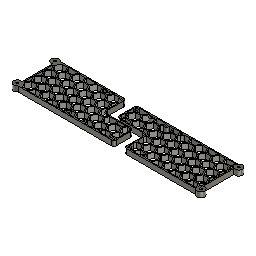
ERCP_Array_Support_Plate_350 (Autodesk Fusion 360 design; units mm, degrees)
Autodesk Fusion 360 part; units mm, degrees
(part 1 of 2)
sketch "Sketch1" plane through (0, 0, 0) normal (0, 0, 1) x (1, 0, 0)
  line L0 (0, 0) -> (490, 0) construction
  line L1 (490, 0) -> (490, 101) construction
  line L2 (490, 101) -> (0, 101) construction
  line L3 (0, 101) -> (0, 0) construction
  circle A0 centre (0, 101) radius 10
  circle A1 centre (0, 0) radius 10
  circle A2 centre (490, 101) radius 10
  circle A3 centre (490, 0) radius 10
  line L4 (0, 50.5) -> (490, 50.5) construction
  circle A4 centre (137.5, 101) radius 2.175
  circle A5 centre (137.5, 101) radius 6
  line L5 (0, 50.5) -> (23.3827, 37) construction
  line L6 (0, 50.5) -> (36.3739, 50.5) construction
  line L7 (23.3827, 37) -> (0, 23.5) construction
  line L8 (23.3827, 37) -> (42.9186, 37) construction
  line L9 (0, 23.5) -> (23.3827, 10) construction
  line L10 (0, 23.5) -> (20, 23.5) construction
  line L11 (211.5, 101) -> (211.5, 63)
  line L12 (263.5, 0) -> (263.5, 38)
  line L13 (183.5, 101) -> (183.5, 58)
  line L14 (291.5, 43) -> (291.5, 0)
  circle A6 centre (0, 0) radius 3
  circle A7 centre (0, 101) radius 3
  circle A8 centre (490, 0) radius 3
  circle A9 centre (490, 101) radius 3
  line L15 (8, 107) -> (177.5, 107)
  line L16 (217.5, 107) -> (482, 107)
  line L17 (482, -6) -> (297.5, -6)
  line L18 (257.5, -6) -> (8, -6)
  line L19 (221.5, 53) -> (281.5, 53)
  line L20 (193.5, 48) -> (253.5, 48)
  arc A10 (183.5, 58) -> (193.5, 48) centre (193.5, 58) ccw
  arc A11 (211.5, 63) -> (221.5, 53) centre (221.5, 63) ccw
  arc A12 (291.5, 43) -> (281.5, 53) centre (281.5, 43) ccw
  arc A13 (263.5, 38) -> (253.5, 48) centre (253.5, 38) ccw
  circle A14 centre (137.5, 0) radius 6
  circle A15 centre (137.5, 0) radius 2.175
  circle A16 centre (177.5, 101) radius 6
  circle A17 centre (177.5, 101) radius 2.175
  circle A18 centre (217.5, 101) radius 6
  circle A19 centre (217.5, 101) radius 2.175
  circle A20 centre (257.5, 101) radius 6
  circle A21 centre (257.5, 101) radius 2.175
  circle A22 centre (297.5, 101) radius 6
  circle A23 centre (297.5, 101) radius 2.175
  circle A24 centre (337.5, 101) radius 6
  circle A25 centre (337.5, 101) radius 2.175
  circle A26 centre (177.5, 0) radius 6
  circle A27 centre (177.5, 0) radius 2.175
  circle A28 centre (217.5, 0) radius 6
  circle A29 centre (217.5, 0) radius 2.175
  circle A30 centre (257.5, 0) radius 6
  circle A31 centre (257.5, 0) radius 2.175
  circle A32 centre (297.5, 0) radius 6
  circle A33 centre (297.5, 0) radius 2.175
  circle A34 centre (337.5, 0) radius 6
  circle A35 centre (337.5, 0) radius 2.175
  line L21 (181, 101) -> (181, 58)
  arc A36 (181, 58) -> (193.5, 45.5) centre (193.5, 58) ccw
  line L22 (193.5, 45.5) -> (253.5, 45.5)
  arc A37 (261, 38) -> (253.5, 45.5) centre (253.5, 38) ccw
  line L23 (261, 0) -> (261, 38)
  line L24 (214, 101) -> (214, 63)
  arc A38 (214, 63) -> (221.5, 55.5) centre (221.5, 63) ccw
  line L25 (221.5, 55.5) -> (281.5, 55.5)
  arc A39 (294, 43) -> (281.5, 55.5) centre (281.5, 43) ccw
  line L26 (294, 43) -> (294, 0)
  line L27 (8, 104.5) -> (177.5, 104.5)
  line L28 (257.5, -3.5) -> (8, -3.5)
  line L29 (482, -3.5) -> (297.5, -3.5)
  line L30 (217.5, 104.5) -> (482, 104.5)
  line L31 (6.9282, 38.5) -> (13.8564, 50.5)
  line L32 (13.8564, 50.5) -> (6.9282, 62.5)
  line L33 (6.9282, 62.5) -> (-6.9282, 62.5)
  line L34 (-6.9282, 62.5) -> (-13.8564, 50.5)
  line L35 (-13.8564, 50.5) -> (-6.9282, 38.5)
  line L36 (-6.9282, 38.5) -> (6.9282, 38.5)
  line L37 (30.3109, 25) -> (37.2391, 37)
  line L38 (37.2391, 37) -> (30.3109, 49)
  line L39 (30.3109, 49) -> (16.4545, 49)
  line L40 (16.4545, 49) -> (9.5263, 37)
  line L41 (9.5263, 37) -> (16.4545, 25)
  line L42 (16.4545, 25) -> (30.3109, 25)
  line L43 (-6.9282, 35.5) -> (-13.8564, 23.5)
  line L44 (-13.8564, 23.5) -> (-6.9282, 11.5)
  line L45 (-6.9282, 11.5) -> (6.9282, 11.5)
  line L46 (6.9282, 11.5) -> (13.8564, 23.5)
  line L47 (13.8564, 23.5) -> (6.9282, 35.5)
  line L48 (6.9282, 35.5) -> (-6.9282, 35.5)
  line L49 (16.4545, 22) -> (9.5263, 10)
  line L50 (9.5263, 10) -> (16.4545, -2)
  line L51 (16.4545, -2) -> (30.3109, -2)
  line L52 (30.3109, -2) -> (37.2391, 10)
  line L53 (37.2391, 10) -> (30.3109, 22)
  line L54 (30.3109, 22) -> (16.4545, 22)
  line L55 (6.9282, 65.5) -> (13.8564, 77.5)
  line L56 (13.8564, 77.5) -> (6.9282, 89.5)
  line L57 (6.9282, 89.5) -> (-6.9282, 89.5)
  line L58 (-6.9282, 89.5) -> (-13.8564, 77.5)
  line L59 (-13.8564, 77.5) -> (-6.9282, 65.5)
  line L60 (-6.9282, 65.5) -> (6.9282, 65.5)
  line L61 (3, 101) -> (3, 0)
  line L62 (487, 101) -> (487, 0)
  line L63 (484, 101) -> (484, 0)
  line L64 (6, 101) -> (6, 0)
  line L65 (137.5, 101) -> (137.5, 146) construction
  line L66 (145, 131) -> (130, 131) construction
  line L67 (130, 131) -> (130, 161) construction
  line L68 (130, 161) -> (145, 161) construction
  line L69 (145, 161) -> (145, 131) construction
  line L70 (145, 131) -> (130, 161) construction
  line L71 (130, 131) -> (145, 161) construction
  line L72 (125, 161) -> (165, 161) construction
  line L73 (165, 161) -> (165, 131) construction
  line L74 (165, 131) -> (125, 131) construction
  line L75 (125, 131) -> (125, 161) construction
  line L76 (125, 181) -> (365, 181) construction
  line L77 (365, 181) -> (365, 151) construction
  line L78 (365, 151) -> (125, 151) construction
  line L79 (125, 151) -> (125, 181) construction
  line L80 (245, 181) -> (245, 151) construction
  line L81 (32.909, 23.5) -> (39.8372, 11.5)
  line L82 (39.8372, 35.5) -> (32.909, 23.5)
  line L83 (53.6936, 35.5) -> (39.8372, 35.5)
  line L84 (60.6218, 23.5) -> (53.6936, 35.5)
  line L85 (53.6936, 11.5) -> (60.6218, 23.5)
  line L86 (63.2199, 22) -> (56.2917, 10)
  line L87 (39.8372, 11.5) -> (53.6936, 11.5)
  line L88 (53.6936, 8.5) -> (39.8372, 8.5)
  line L89 (60.6218, -3.5) -> (53.6936, 8.5)
  line L90 (53.6936, -15.5) -> (60.6218, -3.5)
  line L91 (39.8372, -15.5) -> (53.6936, -15.5)
  line L92 (32.909, -3.5) -> (39.8372, -15.5)
  line L93 (39.8372, 8.5) -> (32.909, -3.5)
  line L94 (77.0763, 22) -> (63.2199, 22)
  line L95 (56.2917, 10) -> (63.2199, -2)
  line L96 (63.2199, -2) -> (77.0763, -2)
  line L97 (77.0763, -2) -> (84.0045, 10)
  line L98 (84.0045, 10) -> (77.0763, 22)
  line L99 (77.0763, -5) -> (63.2199, -5)
  line L100 (63.2199, -5) -> (56.2917, -17)
  line L101 (56.2917, -17) -> (63.2199, -29)
  line L102 (63.2199, -29) -> (77.0763, -29)
  line L103 (77.0763, -29) -> (84.0045, -17)
  line L104 (84.0045, -17) -> (77.0763, -5)
  line L105 (79.6743, -3.5) -> (86.6025, -15.5)
  line L106 (86.6025, 8.5) -> (79.6743, -3.5)
  line L107 (100.4589, 8.5) -> (86.6025, 8.5)
  line L108 (107.3872, -3.5) -> (100.4589, 8.5)
  line L109 (100.4589, -15.5) -> (107.3872, -3.5)
  line L110 (109.9852, -5) -> (103.057, -17)
  line L111 (86.6025, -15.5) -> (100.4589, -15.5)
  line L112 (100.4589, -18.5) -> (86.6025, -18.5)
  line L113 (107.3872, -30.5) -> (100.4589, -18.5)
  line L114 (100.4589, -42.5) -> (107.3872, -30.5)
  line L115 (86.6025, -42.5) -> (100.4589, -42.5)
  line L116 (79.6743, -30.5) -> (86.6025, -42.5)
  line L117 (86.6025, -18.5) -> (79.6743, -30.5)
  line L118 (123.8416, -5) -> (109.9852, -5)
  line L119 (103.057, -17) -> (109.9852, -29)
  line L120 (109.9852, -29) -> (123.8416, -29)
  line L121 (123.8416, -29) -> (130.7698, -17)
  line L122 (130.7698, -17) -> (123.8416, -5)
  line L123 (123.8416, -32) -> (109.9852, -32)
  line L124 (109.9852, -32) -> (103.057, -44)
  line L125 (103.057, -44) -> (109.9852, -56)
  line L126 (109.9852, -56) -> (123.8416, -56)
  line L127 (123.8416, -56) -> (130.7698, -44)
  line L128 (130.7698, -44) -> (123.8416, -32)
  line L129 (126.4397, -30.5) -> (133.3679, -42.5)
  line L130 (133.3679, -18.5) -> (126.4397, -30.5)
  line L131 (147.2243, -18.5) -> (133.3679, -18.5)
  line L132 (154.1525, -30.5) -> (147.2243, -18.5)
  line L133 (147.2243, -42.5) -> (154.1525, -30.5)
  line L134 (156.7506, -32) -> (149.8224, -44)
  line L135 (133.3679, -42.5) -> (147.2243, -42.5)
  line L136 (147.2243, -45.5) -> (133.3679, -45.5)
  line L137 (154.1525, -57.5) -> (147.2243, -45.5)
  line L138 (147.2243, -69.5) -> (154.1525, -57.5)
  line L139 (133.3679, -69.5) -> (147.2243, -69.5)
  line L140 (126.4397, -57.5) -> (133.3679, -69.5)
  line L141 (133.3679, -45.5) -> (126.4397, -57.5)
  line L142 (170.607, -32) -> (156.7506, -32)
  line L143 (149.8224, -44) -> (156.7506, -56)
  line L144 (156.7506, -56) -> (170.607, -56)
  line L145 (170.607, -56) -> (177.5352, -44)
  line L146 (177.5352, -44) -> (170.607, -32)
  line L147 (170.607, -59) -> (156.7506, -59)
  line L148 (156.7506, -59) -> (149.8224, -71)
  line L149 (149.8224, -71) -> (156.7506, -83)
  line L150 (156.7506, -83) -> (170.607, -83)
  line L151 (170.607, -83) -> (177.5352, -71)
  line L152 (177.5352, -71) -> (170.607, -59)
  line L153 (173.2051, -57.5) -> (180.1333, -69.5)
  line L154 (180.1333, -45.5) -> (173.2051, -57.5)
  line L155 (193.9897, -45.5) -> (180.1333, -45.5)
  line L156 (200.9179, -57.5) -> (193.9897, -45.5)
  line L157 (193.9897, -69.5) -> (200.9179, -57.5)
  line L158 (203.516, -59) -> (196.5878, -71)
  line L159 (180.1333, -69.5) -> (193.9897, -69.5)
  line L160 (193.9897, -72.5) -> (180.1333, -72.5)
  line L161 (200.9179, -84.5) -> (193.9897, -72.5)
  line L162 (193.9897, -96.5) -> (200.9179, -84.5)
  line L163 (180.1333, -96.5) -> (193.9897, -96.5)
  line L164 (173.2051, -84.5) -> (180.1333, -96.5)
  line L165 (180.1333, -72.5) -> (173.2051, -84.5)
  line L166 (217.3724, -59) -> (203.516, -59)
  line L167 (196.5878, -71) -> (203.516, -83)
  line L168 (203.516, -83) -> (217.3724, -83)
  line L169 (217.3724, -83) -> (224.3006, -71)
  line L170 (224.3006, -71) -> (217.3724, -59)
  line L171 (217.3724, -86) -> (203.516, -86)
  line L172 (203.516, -86) -> (196.5878, -98)
  line L173 (196.5878, -98) -> (203.516, -110)
  line L174 (203.516, -110) -> (217.3724, -110)
  line L175 (217.3724, -110) -> (224.3006, -98)
  line L176 (224.3006, -98) -> (217.3724, -86)
  line L177 (219.9705, -84.5) -> (226.8987, -96.5)
  line L178 (226.8987, -72.5) -> (219.9705, -84.5)
  line L179 (240.7551, -72.5) -> (226.8987, -72.5)
  line L180 (247.6833, -84.5) -> (240.7551, -72.5)
  line L181 (240.7551, -96.5) -> (247.6833, -84.5)
  line L182 (250.2813, -86) -> (243.3531, -98)
  line L183 (226.8987, -96.5) -> (240.7551, -96.5)
  line L184 (240.7551, -99.5) -> (226.8987, -99.5)
  line L185 (247.6833, -111.5) -> (240.7551, -99.5)
  line L186 (240.7551, -123.5) -> (247.6833, -111.5)
  line L187 (226.8987, -123.5) -> (240.7551, -123.5)
  line L188 (219.9705, -111.5) -> (226.8987, -123.5)
  line L189 (226.8987, -99.5) -> (219.9705, -111.5)
  line L190 (264.1377, -86) -> (250.2813, -86)
  line L191 (243.3531, -98) -> (250.2813, -110)
  line L192 (250.2813, -110) -> (264.1377, -110)
  line L193 (264.1377, -110) -> (271.066, -98)
  line L194 (271.066, -98) -> (264.1377, -86)
  line L195 (264.1377, -113) -> (250.2813, -113)
  line L196 (250.2813, -113) -> (243.3531, -125)
  line L197 (243.3531, -125) -> (250.2813, -137)
  line L198 (250.2813, -137) -> (264.1377, -137)
  line L199 (264.1377, -137) -> (271.066, -125)
  line L200 (271.066, -125) -> (264.1377, -113)
  line L201 (266.7358, -111.5) -> (273.664, -123.5)
  line L202 (273.664, -99.5) -> (266.7358, -111.5)
  line L203 (287.5204, -99.5) -> (273.664, -99.5)
  line L204 (294.4486, -111.5) -> (287.5204, -99.5)
  line L205 (287.5204, -123.5) -> (294.4486, -111.5)
  line L206 (297.0467, -113) -> (290.1185, -125)
  line L207 (273.664, -123.5) -> (287.5204, -123.5)
  line L208 (287.5204, -126.5) -> (273.664, -126.5)
  line L209 (294.4486, -138.5) -> (287.5204, -126.5)
  line L210 (287.5204, -150.5) -> (294.4486, -138.5)
  line L211 (273.664, -150.5) -> (287.5204, -150.5)
  line L212 (266.7358, -138.5) -> (273.664, -150.5)
  line L213 (273.664, -126.5) -> (266.7358, -138.5)
  line L214 (310.9031, -113) -> (297.0467, -113)
  line L215 (290.1185, -125) -> (297.0467, -137)
  line L216 (297.0467, -137) -> (310.9031, -137)
  line L217 (310.9031, -137) -> (317.8313, -125)
  line L218 (317.8313, -125) -> (310.9031, -113)
  line L219 (310.9031, -140) -> (297.0467, -140)
  line L220 (297.0467, -140) -> (290.1185, -152)
  line L221 (290.1185, -152) -> (297.0467, -164)
  line L222 (297.0467, -164) -> (310.9031, -164)
  line L223 (310.9031, -164) -> (317.8313, -152)
  line L224 (317.8313, -152) -> (310.9031, -140)
  line L225 (313.5012, -138.5) -> (320.4294, -150.5)
  line L226 (320.4294, -126.5) -> (313.5012, -138.5)
  line L227 (334.2858, -126.5) -> (320.4294, -126.5)
  line L228 (341.214, -138.5) -> (334.2858, -126.5)
  line L229 (334.2858, -150.5) -> (341.214, -138.5)
  line L230 (343.8121, -140) -> (336.8839, -152)
  line L231 (320.4294, -150.5) -> (334.2858, -150.5)
  line L232 (334.2858, -153.5) -> (320.4294, -153.5)
  line L233 (341.214, -165.5) -> (334.2858, -153.5)
  line L234 (334.2858, -177.5) -> (341.214, -165.5)
  line L235 (320.4294, -177.5) -> (334.2858, -177.5)
  line L236 (313.5012, -165.5) -> (320.4294, -177.5)
  line L237 (320.4294, -153.5) -> (313.5012, -165.5)
  line L238 (357.6685, -140) -> (343.8121, -140)
  line L239 (336.8839, -152) -> (343.8121, -164)
  line L240 (343.8121, -164) -> (357.6685, -164)
  line L241 (357.6685, -164) -> (364.5967, -152)
  line L242 (364.5967, -152) -> (357.6685, -140)
  line L243 (357.6685, -167) -> (343.8121, -167)
  line L244 (343.8121, -167) -> (336.8839, -179)
  line L245 (336.8839, -179) -> (343.8121, -191)
  line L246 (343.8121, -191) -> (357.6685, -191)
  line L247 (357.6685, -191) -> (364.5967, -179)
  line L248 (364.5967, -179) -> (357.6685, -167)
  line L249 (360.2666, -165.5) -> (367.1948, -177.5)
  line L250 (367.1948, -153.5) -> (360.2666, -165.5)
  line L251 (381.0512, -153.5) -> (367.1948, -153.5)
  line L252 (387.9794, -165.5) -> (381.0512, -153.5)
  line L253 (381.0512, -177.5) -> (387.9794, -165.5)
  line L254 (390.5775, -167) -> (383.6493, -179)
  line L255 (367.1948, -177.5) -> (381.0512, -177.5)
  line L256 (381.0512, -180.5) -> (367.1948, -180.5)
  line L257 (387.9794, -192.5) -> (381.0512, -180.5)
  line L258 (381.0512, -204.5) -> (387.9794, -192.5)
  line L259 (367.1948, -204.5) -> (381.0512, -204.5)
  line L260 (360.2666, -192.5) -> (367.1948, -204.5)
  line L261 (367.1948, -180.5) -> (360.2666, -192.5)
  line L262 (404.4339, -167) -> (390.5775, -167)
  line L263 (383.6493, -179) -> (390.5775, -191)
  line L264 (390.5775, -191) -> (404.4339, -191)
  line L265 (404.4339, -191) -> (411.3621, -179)
  line L266 (411.3621, -179) -> (404.4339, -167)
  line L267 (404.4339, -194) -> (390.5775, -194)
  line L268 (390.5775, -194) -> (383.6493, -206)
  line L269 (383.6493, -206) -> (390.5775, -218)
  line L270 (390.5775, -218) -> (404.4339, -218)
  line L271 (404.4339, -218) -> (411.3621, -206)
  line L272 (411.3621, -206) -> (404.4339, -194)
  line L273 (9.5236, 90.9953) -> (16.4518, 78.9953)
  line L274 (16.4518, 102.9953) -> (9.5236, 90.9953)
  line L275 (30.3082, 102.9953) -> (16.4518, 102.9953)
  line L276 (37.2364, 90.9953) -> (30.3082, 102.9953)
  line L277 (30.3082, 78.9953) -> (37.2364, 90.9953)
  line L278 (39.8345, 89.4953) -> (32.9063, 77.4953)
  line L279 (16.4518, 78.9953) -> (30.3082, 78.9953)
  line L280 (30.3082, 75.9953) -> (16.4518, 75.9953)
  line L281 (37.2364, 63.9953) -> (30.3082, 75.9953)
  line L282 (30.3082, 51.9953) -> (37.2364, 63.9953)
  line L283 (16.4518, 51.9953) -> (30.3082, 51.9953)
  line L284 (9.5236, 63.9953) -> (16.4518, 51.9953)
  line L285 (16.4518, 75.9953) -> (9.5236, 63.9953)
  line L286 (53.6909, 89.4953) -> (39.8345, 89.4953)
  line L287 (32.9063, 77.4953) -> (39.8345, 65.4953)
  line L288 (39.8345, 65.4953) -> (53.6909, 65.4953)
  line L289 (53.6909, 65.4953) -> (60.6191, 77.4953)
  line L290 (60.6191, 77.4953) -> (53.6909, 89.4953)
  line L291 (53.6909, 62.4953) -> (39.8345, 62.4953)
  line L292 (39.8345, 62.4953) -> (32.9063, 50.4953)
  line L293 (32.9063, 50.4953) -> (39.8345, 38.4953)
  line L294 (39.8345, 38.4953) -> (53.6909, 38.4953)
  line L295 (53.6909, 38.4953) -> (60.6191, 50.4953)
  line L296 (60.6191, 50.4953) -> (53.6909, 62.4953)
  line L297 (56.289, 63.9953) -> (63.2172, 51.9953)
  line L298 (63.2172, 75.9953) -> (56.289, 63.9953)
  line L299 (77.0736, 75.9953) -> (63.2172, 75.9953)
  line L300 (84.0018, 63.9953) -> (77.0736, 75.9953)
  line L301 (77.0736, 51.9953) -> (84.0018, 63.9953)
  line L302 (86.5999, 62.4953) -> (79.6717, 50.4953)
  line L303 (63.2172, 51.9953) -> (77.0736, 51.9953)
  line L304 (77.0736, 48.9953) -> (63.2172, 48.9953)
  line L305 (84.0018, 36.9953) -> (77.0736, 48.9953)
  line L306 (77.0736, 24.9953) -> (84.0018, 36.9953)
  line L307 (63.2172, 24.9953) -> (77.0736, 24.9953)
  line L308 (56.289, 36.9953) -> (63.2172, 24.9953)
  line L309 (63.2172, 48.9953) -> (56.289, 36.9953)
  line L310 (100.4563, 62.4953) -> (86.5999, 62.4953)
  line L311 (79.6717, 50.4953) -> (86.5999, 38.4953)
  line L312 (86.5999, 38.4953) -> (100.4563, 38.4953)
  line L313 (100.4563, 38.4953) -> (107.3845, 50.4953)
  line L314 (107.3845, 50.4953) -> (100.4563, 62.4953)
  line L315 (100.4563, 35.4953) -> (86.5999, 35.4953)
  line L316 (86.5999, 35.4953) -> (79.6717, 23.4953)
  line L317 (79.6717, 23.4953) -> (86.5999, 11.4953)
  line L318 (86.5999, 11.4953) -> (100.4563, 11.4953)
  line L319 (100.4563, 11.4953) -> (107.3845, 23.4953)
  line L320 (107.3845, 23.4953) -> (100.4563, 35.4953)
  line L321 (103.0543, 36.9953) -> (109.9825, 24.9953)
  line L322 (109.9825, 48.9953) -> (103.0543, 36.9953)
  line L323 (123.8389, 48.9953) -> (109.9825, 48.9953)
  line L324 (130.7672, 36.9953) -> (123.8389, 48.9953)
  line L325 (123.8389, 24.9953) -> (130.7672, 36.9953)
  line L326 (133.3652, 35.4953) -> (126.437, 23.4953)
  line L327 (109.9825, 24.9953) -> (123.8389, 24.9953)
  line L328 (123.8389, 21.9953) -> (109.9825, 21.9953)
  line L329 (130.7672, 9.9953) -> (123.8389, 21.9953)
  line L330 (123.8389, -2.0047) -> (130.7672, 9.9953)
  line L331 (109.9825, -2.0047) -> (123.8389, -2.0047)
  line L332 (103.0543, 9.9953) -> (109.9825, -2.0047)
  line L333 (109.9825, 21.9953) -> (103.0543, 9.9953)
  line L334 (147.2216, 35.4953) -> (133.3652, 35.4953)
  line L335 (126.437, 23.4953) -> (133.3652, 11.4953)
  line L336 (133.3652, 11.4953) -> (147.2216, 11.4953)
  line L337 (147.2216, 11.4953) -> (154.1498, 23.4953)
  line L338 (154.1498, 23.4953) -> (147.2216, 35.4953)
  line L339 (147.2216, 8.4953) -> (133.3652, 8.4953)
  line L340 (133.3652, 8.4953) -> (126.437, -3.5047)
  line L341 (126.437, -3.5047) -> (133.3652, -15.5047)
  line L342 (133.3652, -15.5047) -> (147.2216, -15.5047)
  line L343 (147.2216, -15.5047) -> (154.1498, -3.5047)
  line L344 (154.1498, -3.5047) -> (147.2216, 8.4953)
  line L345 (149.8197, 9.9953) -> (156.7479, -2.0047)
  line L346 (156.7479, 21.9953) -> (149.8197, 9.9953)
  line L347 (170.6043, 21.9953) -> (156.7479, 21.9953)
  line L348 (177.5325, 9.9953) -> (170.6043, 21.9953)
  line L349 (170.6043, -2.0047) -> (177.5325, 9.9953)
  line L350 (180.1306, 8.4953) -> (173.2024, -3.5047)
  line L351 (156.7479, -2.0047) -> (170.6043, -2.0047)
  line L352 (170.6043, -5.0047) -> (156.7479, -5.0047)
  line L353 (177.5325, -17.0047) -> (170.6043, -5.0047)
  line L354 (170.6043, -29.0047) -> (177.5325, -17.0047)
  line L355 (156.7479, -29.0047) -> (170.6043, -29.0047)
  line L356 (149.8197, -17.0047) -> (156.7479, -29.0047)
  line L357 (156.7479, -5.0047) -> (149.8197, -17.0047)
  line L358 (193.987, 8.4953) -> (180.1306, 8.4953)
  line L359 (173.2024, -3.5047) -> (180.1306, -15.5047)
  line L360 (180.1306, -15.5047) -> (193.987, -15.5047)
  line L361 (193.987, -15.5047) -> (200.9152, -3.5047)
  line L362 (200.9152, -3.5047) -> (193.987, 8.4953)
  line L363 (193.987, -18.5047) -> (180.1306, -18.5047)
  line L364 (180.1306, -18.5047) -> (173.2024, -30.5047)
  line L365 (173.2024, -30.5047) -> (180.1306, -42.5047)
  line L366 (180.1306, -42.5047) -> (193.987, -42.5047)
  line L367 (193.987, -42.5047) -> (200.9152, -30.5047)
  line L368 (200.9152, -30.5047) -> (193.987, -18.5047)
  line L369 (196.5851, -17.0047) -> (203.5133, -29.0047)
  line L370 (203.5133, -5.0047) -> (196.5851, -17.0047)
  line L371 (217.3697, -5.0047) -> (203.5133, -5.0047)
  line L372 (224.2979, -17.0047) -> (217.3697, -5.0047)
  line L373 (217.3697, -29.0047) -> (224.2979, -17.0047)
  line L374 (226.896, -18.5047) -> (219.9678, -30.5047)
  line L375 (203.5133, -29.0047) -> (217.3697, -29.0047)
  line L376 (217.3697, -32.0047) -> (203.5133, -32.0047)
  line L377 (224.2979, -44.0047) -> (217.3697, -32.0047)
  line L378 (217.3697, -56.0047) -> (224.2979, -44.0047)
  line L379 (203.5133, -56.0047) -> (217.3697, -56.0047)
  line L380 (196.5851, -44.0047) -> (203.5133, -56.0047)
  line L381 (203.5133, -32.0047) -> (196.5851, -44.0047)
  line L382 (240.7524, -18.5047) -> (226.896, -18.5047)
  line L383 (219.9678, -30.5047) -> (226.896, -42.5047)
  line L384 (226.896, -42.5047) -> (240.7524, -42.5047)
  line L385 (240.7524, -42.5047) -> (247.6806, -30.5047)
  line L386 (247.6806, -30.5047) -> (240.7524, -18.5047)
  line L387 (240.7524, -45.5047) -> (226.896, -45.5047)
  line L388 (226.896, -45.5047) -> (219.9678, -57.5047)
  line L389 (219.9678, -57.5047) -> (226.896, -69.5047)
  line L390 (226.896, -69.5047) -> (240.7524, -69.5047)
  line L391 (240.7524, -69.5047) -> (247.6806, -57.5047)
  line L392 (247.6806, -57.5047) -> (240.7524, -45.5047)
  line L393 (243.3505, -44.0047) -> (250.2787, -56.0047)
  line L394 (250.2787, -32.0047) -> (243.3505, -44.0047)
  line L395 (264.1351, -32.0047) -> (250.2787, -32.0047)
  line L396 (271.0633, -44.0047) -> (264.1351, -32.0047)
  line L397 (264.1351, -56.0047) -> (271.0633, -44.0047)
  line L398 (273.6613, -45.5047) -> (266.7331, -57.5047)
  line L399 (250.2787, -56.0047) -> (264.1351, -56.0047)
  line L400 (264.1351, -59.0047) -> (250.2787, -59.0047)
  line L401 (271.0633, -71.0047) -> (264.1351, -59.0047)
  line L402 (264.1351, -83.0047) -> (271.0633, -71.0047)
  line L403 (250.2787, -83.0047) -> (264.1351, -83.0047)
  line L404 (243.3505, -71.0047) -> (250.2787, -83.0047)
  line L405 (250.2787, -59.0047) -> (243.3505, -71.0047)
  line L406 (287.5177, -45.5047) -> (273.6613, -45.5047)
  line L407 (266.7331, -57.5047) -> (273.6613, -69.5047)
  line L408 (273.6613, -69.5047) -> (287.5177, -69.5047)
  line L409 (287.5177, -69.5047) -> (294.446, -57.5047)
  line L410 (294.446, -57.5047) -> (287.5177, -45.5047)
  line L411 (287.5177, -72.5047) -> (273.6613, -72.5047)
  line L412 (273.6613, -72.5047) -> (266.7331, -84.5047)
  line L413 (266.7331, -84.5047) -> (273.6613, -96.5047)
  line L414 (273.6613, -96.5047) -> (287.5177, -96.5047)
  line L415 (287.5177, -96.5047) -> (294.446, -84.5047)
  line L416 (294.446, -84.5047) -> (287.5177, -72.5047)
  line L417 (290.1158, -71.0047) -> (297.044, -83.0047)
  line L418 (297.044, -59.0047) -> (290.1158, -71.0047)
  line L419 (310.9004, -59.0047) -> (297.044, -59.0047)
  line L420 (317.8286, -71.0047) -> (310.9004, -59.0047)
  line L421 (310.9004, -83.0047) -> (317.8286, -71.0047)
  line L422 (320.4267, -72.5047) -> (313.4985, -84.5047)
  line L423 (297.044, -83.0047) -> (310.9004, -83.0047)
  line L424 (310.9004, -86.0047) -> (297.044, -86.0047)
  line L425 (317.8286, -98.0047) -> (310.9004, -86.0047)
  line L426 (310.9004, -110.0047) -> (317.8286, -98.0047)
  line L427 (297.044, -110.0047) -> (310.9004, -110.0047)
  line L428 (290.1158, -98.0047) -> (297.044, -110.0047)
  line L429 (297.044, -86.0047) -> (290.1158, -98.0047)
  line L430 (334.2831, -72.5047) -> (320.4267, -72.5047)
  line L431 (313.4985, -84.5047) -> (320.4267, -96.5047)
  line L432 (320.4267, -96.5047) -> (334.2831, -96.5047)
  line L433 (334.2831, -96.5047) -> (341.2113, -84.5047)
  line L434 (341.2113, -84.5047) -> (334.2831, -72.5047)
  line L435 (334.2831, -99.5047) -> (320.4267, -99.5047)
  line L436 (320.4267, -99.5047) -> (313.4985, -111.5047)
  line L437 (313.4985, -111.5047) -> (320.4267, -123.5047)
  line L438 (320.4267, -123.5047) -> (334.2831, -123.5047)
  line L439 (334.2831, -123.5047) -> (341.2113, -111.5047)
  line L440 (341.2113, -111.5047) -> (334.2831, -99.5047)
  line L441 (336.8812, -98.0047) -> (343.8094, -110.0047)
  line L442 (343.8094, -86.0047) -> (336.8812, -98.0047)
  line L443 (357.6658, -86.0047) -> (343.8094, -86.0047)
  line L444 (364.594, -98.0047) -> (357.6658, -86.0047)
  line L445 (357.6658, -110.0047) -> (364.594, -98.0047)
  line L446 (367.1921, -99.5047) -> (360.2639, -111.5047)
  line L447 (343.8094, -110.0047) -> (357.6658, -110.0047)
  line L448 (357.6658, -113.0047) -> (343.8094, -113.0047)
  line L449 (364.594, -125.0047) -> (357.6658, -113.0047)
  line L450 (357.6658, -137.0047) -> (364.594, -125.0047)
  line L451 (343.8094, -137.0047) -> (357.6658, -137.0047)
  line L452 (336.8812, -125.0047) -> (343.8094, -137.0047)
  line L453 (343.8094, -113.0047) -> (336.8812, -125.0047)
  line L454 (381.0485, -99.5047) -> (367.1921, -99.5047)
  line L455 (360.2639, -111.5047) -> (367.1921, -123.5047)
  line L456 (367.1921, -123.5047) -> (381.0485, -123.5047)
  line L457 (381.0485, -123.5047) -> (387.9767, -111.5047)
  line L458 (387.9767, -111.5047) -> (381.0485, -99.5047)
  line L459 (381.0485, -126.5047) -> (367.1921, -126.5047)
  line L460 (367.1921, -126.5047) -> (360.2639, -138.5047)
  line L461 (360.2639, -138.5047) -> (367.1921, -150.5047)
  line L462 (367.1921, -150.5047) -> (381.0485, -150.5047)
  line L463 (381.0485, -150.5047) -> (387.9767, -138.5047)
  line L464 (387.9767, -138.5047) -> (381.0485, -126.5047)
  line L465 (383.6466, -125.0047) -> (390.5748, -137.0047)
  line L466 (390.5748, -113.0047) -> (383.6466, -125.0047)
  line L467 (404.4312, -113.0047) -> (390.5748, -113.0047)
  line L468 (411.3594, -125.0047) -> (404.4312, -113.0047)
  line L469 (404.4312, -137.0047) -> (411.3594, -125.0047)
  line L470 (413.9575, -126.5047) -> (407.0293, -138.5047)
  line L471 (390.5748, -137.0047) -> (404.4312, -137.0047)
  line L472 (404.4312, -140.0047) -> (390.5748, -140.0047)
  line L473 (411.3594, -152.0047) -> (404.4312, -140.0047)
  line L474 (404.4312, -164.0047) -> (411.3594, -152.0047)
  line L475 (390.5748, -164.0047) -> (404.4312, -164.0047)
  line L476 (383.6466, -152.0047) -> (390.5748, -164.0047)
  line L477 (390.5748, -140.0047) -> (383.6466, -152.0047)
  line L478 (427.8139, -126.5047) -> (413.9575, -126.5047)
  line L479 (407.0293, -138.5047) -> (413.9575, -150.5047)
  line L480 (413.9575, -150.5047) -> (427.8139, -150.5047)
  line L481 (427.8139, -150.5047) -> (434.7421, -138.5047)
  line L482 (434.7421, -138.5047) -> (427.8139, -126.5047)
  line L483 (427.8139, -153.5047) -> (413.9575, -153.5047)
  line L484 (413.9575, -153.5047) -> (407.0293, -165.5047)
  line L485 (407.0293, -165.5047) -> (413.9575, -177.5047)
  line L486 (413.9575, -177.5047) -> (427.8139, -177.5047)
  line L487 (427.8139, -177.5047) -> (434.7421, -165.5047)
  line L488 (434.7421, -165.5047) -> (427.8139, -153.5047)
  line L489 (32.9036, 131.4907) -> (39.8318, 119.4907)
  line L490 (39.8318, 143.4907) -> (32.9036, 131.4907)
  line L491 (53.6882, 143.4907) -> (39.8318, 143.4907)
  line L492 (60.6164, 131.4907) -> (53.6882, 143.4907)
  line L493 (53.6882, 119.4907) -> (60.6164, 131.4907)
  line L494 (63.2145, 129.9907) -> (56.2863, 117.9907)
  line L495 (39.8318, 119.4907) -> (53.6882, 119.4907)
  line L496 (53.6882, 116.4907) -> (39.8318, 116.4907)
  line L497 (60.6164, 104.4907) -> (53.6882, 116.4907)
  line L498 (53.6882, 92.4907) -> (60.6164, 104.4907)
  line L499 (39.8318, 92.4907) -> (53.6882, 92.4907)
  line L500 (32.9036, 104.4907) -> (39.8318, 92.4907)
  line L501 (39.8318, 116.4907) -> (32.9036, 104.4907)
  line L502 (77.0709, 129.9907) -> (63.2145, 129.9907)
  line L503 (56.2863, 117.9907) -> (63.2145, 105.9907)
  line L504 (63.2145, 105.9907) -> (77.0709, 105.9907)
  line L505 (77.0709, 105.9907) -> (83.9991, 117.9907)
  line L506 (83.9991, 117.9907) -> (77.0709, 129.9907)
  line L507 (77.0709, 102.9907) -> (63.2145, 102.9907)
  line L508 (63.2145, 102.9907) -> (56.2863, 90.9907)
  line L509 (56.2863, 90.9907) -> (63.2145, 78.9907)
  line L510 (63.2145, 78.9907) -> (77.0709, 78.9907)
  line L511 (77.0709, 78.9907) -> (83.9991, 90.9907)
  line L512 (83.9991, 90.9907) -> (77.0709, 102.9907)
  line L513 (79.669, 104.4907) -> (86.5972, 92.4907)
  line L514 (86.5972, 116.4907) -> (79.669, 104.4907)
  line L515 (100.4536, 116.4907) -> (86.5972, 116.4907)
  line L516 (107.3818, 104.4907) -> (100.4536, 116.4907)
  line L517 (100.4536, 92.4907) -> (107.3818, 104.4907)
  line L518 (109.9799, 102.9907) -> (103.0517, 90.9907)
  line L519 (86.5972, 92.4907) -> (100.4536, 92.4907)
  line L520 (100.4536, 89.4907) -> (86.5972, 89.4907)
  line L521 (107.3818, 77.4907) -> (100.4536, 89.4907)
  line L522 (100.4536, 65.4907) -> (107.3818, 77.4907)
  line L523 (86.5972, 65.4907) -> (100.4536, 65.4907)
  line L524 (79.669, 77.4907) -> (86.5972, 65.4907)
  line L525 (86.5972, 89.4907) -> (79.669, 77.4907)
  line L526 (123.8363, 102.9907) -> (109.9799, 102.9907)
  line L527 (103.0517, 90.9907) -> (109.9799, 78.9907)
  line L528 (109.9799, 78.9907) -> (123.8363, 78.9907)
  line L529 (123.8363, 78.9907) -> (130.7645, 90.9907)
  line L530 (130.7645, 90.9907) -> (123.8363, 102.9907)
  line L531 (123.8363, 75.9907) -> (109.9799, 75.9907)
  line L532 (109.9799, 75.9907) -> (103.0517, 63.9907)
  line L533 (103.0517, 63.9907) -> (109.9799, 51.9907)
  line L534 (109.9799, 51.9907) -> (123.8363, 51.9907)
  line L535 (123.8363, 51.9907) -> (130.7645, 63.9907)
  line L536 (130.7645, 63.9907) -> (123.8363, 75.9907)
  line L537 (126.4343, 77.4907) -> (133.3625, 65.4907)
  line L538 (133.3625, 89.4907) -> (126.4343, 77.4907)
  line L539 (147.2189, 89.4907) -> (133.3625, 89.4907)
  line L540 (154.1472, 77.4907) -> (147.2189, 89.4907)
  line L541 (147.2189, 65.4907) -> (154.1472, 77.4907)
  line L542 (156.7452, 75.9907) -> (149.817, 63.9907)
  line L543 (133.3625, 65.4907) -> (147.2189, 65.4907)
  line L544 (147.2189, 62.4907) -> (133.3625, 62.4907)
  line L545 (154.1472, 50.4907) -> (147.2189, 62.4907)
  line L546 (147.2189, 38.4907) -> (154.1472, 50.4907)
  line L547 (133.3625, 38.4907) -> (147.2189, 38.4907)
  line L548 (126.4343, 50.4907) -> (133.3625, 38.4907)
  line L549 (133.3625, 62.4907) -> (126.4343, 50.4907)
  line L550 (170.6016, 75.9907) -> (156.7452, 75.9907)
  line L551 (149.817, 63.9907) -> (156.7452, 51.9907)
  line L552 (156.7452, 51.9907) -> (170.6016, 51.9907)
  line L553 (170.6016, 51.9907) -> (177.5298, 63.9907)
  line L554 (177.5298, 63.9907) -> (170.6016, 75.9907)
  line L555 (170.6016, 48.9907) -> (156.7452, 48.9907)
  line L556 (156.7452, 48.9907) -> (149.817, 36.9907)
  line L557 (149.817, 36.9907) -> (156.7452, 24.9907)
  line L558 (156.7452, 24.9907) -> (170.6016, 24.9907)
  line L559 (170.6016, 24.9907) -> (177.5298, 36.9907)
  line L560 (177.5298, 36.9907) -> (170.6016, 48.9907)
  line L561 (173.1997, 50.4907) -> (180.1279, 38.4907)
  line L562 (180.1279, 62.4907) -> (173.1997, 50.4907)
  line L563 (193.9843, 62.4907) -> (180.1279, 62.4907)
  line L564 (200.9125, 50.4907) -> (193.9843, 62.4907)
  line L565 (193.9843, 38.4907) -> (200.9125, 50.4907)
  line L566 (203.5106, 48.9907) -> (196.5824, 36.9907)
  line L567 (180.1279, 38.4907) -> (193.9843, 38.4907)
  line L568 (193.9843, 35.4907) -> (180.1279, 35.4907)
  line L569 (200.9125, 23.4907) -> (193.9843, 35.4907)
  line L570 (193.9843, 11.4907) -> (200.9125, 23.4907)
  line L571 (180.1279, 11.4907) -> (193.9843, 11.4907)
  line L572 (173.1997, 23.4907) -> (180.1279, 11.4907)
  line L573 (180.1279, 35.4907) -> (173.1997, 23.4907)
  line L574 (217.367, 48.9907) -> (203.5106, 48.9907)
  line L575 (196.5824, 36.9907) -> (203.5106, 24.9907)
  line L576 (203.5106, 24.9907) -> (217.367, 24.9907)
  line L577 (217.367, 24.9907) -> (224.2952, 36.9907)
  line L578 (224.2952, 36.9907) -> (217.367, 48.9907)
  line L579 (217.367, 21.9907) -> (203.5106, 21.9907)
  line L580 (203.5106, 21.9907) -> (196.5824, 9.9907)
  line L581 (196.5824, 9.9907) -> (203.5106, -2.0093)
  line L582 (203.5106, -2.0093) -> (217.367, -2.0093)
  line L583 (217.367, -2.0093) -> (224.2952, 9.9907)
  line L584 (224.2952, 9.9907) -> (217.367, 21.9907)
  line L585 (219.9651, 23.4907) -> (226.8933, 11.4907)
  line L586 (226.8933, 35.4907) -> (219.9651, 23.4907)
  line L587 (240.7497, 35.4907) -> (226.8933, 35.4907)
  line L588 (247.6779, 23.4907) -> (240.7497, 35.4907)
  line L589 (240.7497, 11.4907) -> (247.6779, 23.4907)
  line L590 (250.276, 21.9907) -> (243.3478, 9.9907)
  line L591 (226.8933, 11.4907) -> (240.7497, 11.4907)
  line L592 (240.7497, 8.4907) -> (226.8933, 8.4907)
  line L593 (247.6779, -3.5093) -> (240.7497, 8.4907)
  line L594 (240.7497, -15.5093) -> (247.6779, -3.5093)
  line L595 (226.8933, -15.5093) -> (240.7497, -15.5093)
  line L596 (219.9651, -3.5093) -> (226.8933, -15.5093)
  line L597 (226.8933, 8.4907) -> (219.9651, -3.5093)
  line L598 (264.1324, 21.9907) -> (250.276, 21.9907)
  line L599 (243.3478, 9.9907) -> (250.276, -2.0093)
  line L600 (250.276, -2.0093) -> (264.1324, -2.0093)
  line L601 (264.1324, -2.0093) -> (271.0606, 9.9907)
  line L602 (271.0606, 9.9907) -> (264.1324, 21.9907)
  line L603 (264.1324, -5.0093) -> (250.276, -5.0093)
  line L604 (250.276, -5.0093) -> (243.3478, -17.0093)
  line L605 (243.3478, -17.0093) -> (250.276, -29.0093)
  line L606 (250.276, -29.0093) -> (264.1324, -29.0093)
  line L607 (264.1324, -29.0093) -> (271.0606, -17.0093)
  line L608 (271.0606, -17.0093) -> (264.1324, -5.0093)
  line L609 (266.7305, -3.5093) -> (273.6587, -15.5093)
  line L610 (273.6587, 8.4907) -> (266.7305, -3.5093)
  line L611 (287.5151, 8.4907) -> (273.6587, 8.4907)
  line L612 (294.4433, -3.5093) -> (287.5151, 8.4907)
  line L613 (287.5151, -15.5093) -> (294.4433, -3.5093)
  line L614 (297.0413, -5.0093) -> (290.1131, -17.0093)
  line L615 (273.6587, -15.5093) -> (287.5151, -15.5093)
  line L616 (287.5151, -18.5093) -> (273.6587, -18.5093)
  line L617 (294.4433, -30.5093) -> (287.5151, -18.5093)
  line L618 (287.5151, -42.5093) -> (294.4433, -30.5093)
  line L619 (273.6587, -42.5093) -> (287.5151, -42.5093)
  line L620 (266.7305, -30.5093) -> (273.6587, -42.5093)
  line L621 (273.6587, -18.5093) -> (266.7305, -30.5093)
  line L622 (310.8977, -5.0093) -> (297.0413, -5.0093)
  line L623 (290.1131, -17.0093) -> (297.0413, -29.0093)
  line L624 (297.0413, -29.0093) -> (310.8977, -29.0093)
  line L625 (310.8977, -29.0093) -> (317.826, -17.0093)
  line L626 (317.826, -17.0093) -> (310.8977, -5.0093)
  line L627 (310.8977, -32.0093) -> (297.0413, -32.0093)
  line L628 (297.0413, -32.0093) -> (290.1131, -44.0093)
  line L629 (290.1131, -44.0093) -> (297.0413, -56.0093)
  line L630 (297.0413, -56.0093) -> (310.8977, -56.0093)
  line L631 (310.8977, -56.0093) -> (317.826, -44.0093)
  line L632 (317.826, -44.0093) -> (310.8977, -32.0093)
  line L633 (313.4958, -30.5093) -> (320.424, -42.5093)
  line L634 (320.424, -18.5093) -> (313.4958, -30.5093)
  line L635 (334.2804, -18.5093) -> (320.424, -18.5093)
  line L636 (341.2086, -30.5093) -> (334.2804, -18.5093)
  line L637 (334.2804, -42.5093) -> (341.2086, -30.5093)
  line L638 (343.8067, -32.0093) -> (336.8785, -44.0093)
  line L639 (320.424, -42.5093) -> (334.2804, -42.5093)
  line L640 (334.2804, -45.5093) -> (320.424, -45.5093)
  line L641 (341.2086, -57.5093) -> (334.2804, -45.5093)
  line L642 (334.2804, -69.5093) -> (341.2086, -57.5093)
  line L643 (320.424, -69.5093) -> (334.2804, -69.5093)
  line L644 (313.4958, -57.5093) -> (320.424, -69.5093)
  line L645 (320.424, -45.5093) -> (313.4958, -57.5093)
  line L646 (357.6631, -32.0093) -> (343.8067, -32.0093)
  line L647 (336.8785, -44.0093) -> (343.8067, -56.0093)
  line L648 (343.8067, -56.0093) -> (357.6631, -56.0093)
  line L649 (357.6631, -56.0093) -> (364.5913, -44.0093)
  line L650 (364.5913, -44.0093) -> (357.6631, -32.0093)
  line L651 (357.6631, -59.0093) -> (343.8067, -59.0093)
  line L652 (343.8067, -59.0093) -> (336.8785, -71.0093)
  line L653 (336.8785, -71.0093) -> (343.8067, -83.0093)
  line L654 (343.8067, -83.0093) -> (357.6631, -83.0093)
  line L655 (357.6631, -83.0093) -> (364.5913, -71.0093)
  line L656 (364.5913, -71.0093) -> (357.6631, -59.0093)
  line L657 (360.2612, -57.5093) -> (367.1894, -69.5093)
  line L658 (367.1894, -45.5093) -> (360.2612, -57.5093)
  line L659 (381.0458, -45.5093) -> (367.1894, -45.5093)
  line L660 (387.974, -57.5093) -> (381.0458, -45.5093)
  line L661 (381.0458, -69.5093) -> (387.974, -57.5093)
  line L662 (390.5721, -59.0093) -> (383.6439, -71.0093)
  line L663 (367.1894, -69.5093) -> (381.0458, -69.5093)
  line L664 (381.0458, -72.5093) -> (367.1894, -72.5093)
  line L665 (387.974, -84.5093) -> (381.0458, -72.5093)
  line L666 (381.0458, -96.5093) -> (387.974, -84.5093)
  line L667 (367.1894, -96.5093) -> (381.0458, -96.5093)
  line L668 (360.2612, -84.5093) -> (367.1894, -96.5093)
  line L669 (367.1894, -72.5093) -> (360.2612, -84.5093)
  line L670 (404.4285, -59.0093) -> (390.5721, -59.0093)
  line L671 (383.6439, -71.0093) -> (390.5721, -83.0093)
  line L672 (390.5721, -83.0093) -> (404.4285, -83.0093)
  line L673 (404.4285, -83.0093) -> (411.3567, -71.0093)
  line L674 (411.3567, -71.0093) -> (404.4285, -59.0093)
  line L675 (404.4285, -86.0093) -> (390.5721, -86.0093)
  line L676 (390.5721, -86.0093) -> (383.6439, -98.0093)
  line L677 (383.6439, -98.0093) -> (390.5721, -110.0093)
  line L678 (390.5721, -110.0093) -> (404.4285, -110.0093)
  line L679 (404.4285, -110.0093) -> (411.3567, -98.0093)
  line L680 (411.3567, -98.0093) -> (404.4285, -86.0093)
  line L681 (407.0266, -84.5093) -> (413.9548, -96.5093)
  line L682 (413.9548, -72.5093) -> (407.0266, -84.5093)
  line L683 (427.8112, -72.5093) -> (413.9548, -72.5093)
  line L684 (434.7394, -84.5093) -> (427.8112, -72.5093)
  line L685 (427.8112, -96.5093) -> (434.7394, -84.5093)
  line L686 (437.3375, -86.0093) -> (430.4093, -98.0093)
  line L687 (413.9548, -96.5093) -> (427.8112, -96.5093)
  line L688 (427.8112, -99.5093) -> (413.9548, -99.5093)
  line L689 (434.7394, -111.5093) -> (427.8112, -99.5093)
  line L690 (427.8112, -123.5093) -> (434.7394, -111.5093)
  line L691 (413.9548, -123.5093) -> (427.8112, -123.5093)
  line L692 (407.0266, -111.5093) -> (413.9548, -123.5093)
  line L693 (413.9548, -99.5093) -> (407.0266, -111.5093)
  line L694 (451.1939, -86.0093) -> (437.3375, -86.0093)
  line L695 (430.4093, -98.0093) -> (437.3375, -110.0093)
  line L696 (437.3375, -110.0093) -> (451.1939, -110.0093)
  line L697 (451.1939, -110.0093) -> (458.1221, -98.0093)
  line L698 (458.1221, -98.0093) -> (451.1939, -86.0093)
  line L699 (451.1939, -113.0093) -> (437.3375, -113.0093)
  line L700 (437.3375, -113.0093) -> (430.4093, -125.0093)
  line L701 (430.4093, -125.0093) -> (437.3375, -137.0093)
  line L702 (437.3375, -137.0093) -> (451.1939, -137.0093)
  line L703 (451.1939, -137.0093) -> (458.1221, -125.0093)
  line L704 (458.1221, -125.0093) -> (451.1939, -113.0093)
  line L705 (56.2836, 171.986) -> (63.2118, 159.986)
  line L706 (63.2118, 183.986) -> (56.2836, 171.986)
  line L707 (77.0682, 183.986) -> (63.2118, 183.986)
  line L708 (83.9964, 171.986) -> (77.0682, 183.986)
  line L709 (77.0682, 159.986) -> (83.9964, 171.986)
  line L710 (86.5945, 170.486) -> (79.6663, 158.486)
  line L711 (63.2118, 159.986) -> (77.0682, 159.986)
  line L712 (77.0682, 156.986) -> (63.2118, 156.986)
  line L713 (83.9964, 144.986) -> (77.0682, 156.986)
  line L714 (77.0682, 132.986) -> (83.9964, 144.986)
  line L715 (63.2118, 132.986) -> (77.0682, 132.986)
  line L716 (56.2836, 144.986) -> (63.2118, 132.986)
  line L717 (63.2118, 156.986) -> (56.2836, 144.986)
  line L718 (100.4509, 170.486) -> (86.5945, 170.486)
  line L719 (79.6663, 158.486) -> (86.5945, 146.486)
  line L720 (86.5945, 146.486) -> (100.4509, 146.486)
  line L721 (100.4509, 146.486) -> (107.3791, 158.486)
  line L722 (107.3791, 158.486) -> (100.4509, 170.486)
  line L723 (100.4509, 143.486) -> (86.5945, 143.486)
  line L724 (86.5945, 143.486) -> (79.6663, 131.486)
  line L725 (79.6663, 131.486) -> (86.5945, 119.486)
  line L726 (86.5945, 119.486) -> (100.4509, 119.486)
  line L727 (100.4509, 119.486) -> (107.3791, 131.486)
  line L728 (107.3791, 131.486) -> (100.4509, 143.486)
  line L729 (103.049, 144.986) -> (109.9772, 132.986)
  line L730 (109.9772, 156.986) -> (103.049, 144.986)
  line L731 (123.8336, 156.986) -> (109.9772, 156.986)
  line L732 (130.7618, 144.986) -> (123.8336, 156.986)
  line L733 (123.8336, 132.986) -> (130.7618, 144.986)
  line L734 (133.3599, 143.486) -> (126.4317, 131.486)
  line L735 (109.9772, 132.986) -> (123.8336, 132.986)
  line L736 (123.8336, 129.986) -> (109.9772, 129.986)
  line L737 (130.7618, 117.986) -> (123.8336, 129.986)
  line L738 (123.8336, 105.986) -> (130.7618, 117.986)
  line L739 (109.9772, 105.986) -> (123.8336, 105.986)
  line L740 (103.049, 117.986) -> (109.9772, 105.986)
  line L741 (109.9772, 129.986) -> (103.049, 117.986)
  line L742 (147.2163, 143.486) -> (133.3599, 143.486)
  line L743 (126.4317, 131.486) -> (133.3599, 119.486)
  line L744 (133.3599, 119.486) -> (147.2163, 119.486)
  line L745 (147.2163, 119.486) -> (154.1445, 131.486)
  line L746 (154.1445, 131.486) -> (147.2163, 143.486)
  line L747 (147.2163, 116.486) -> (133.3599, 116.486)
  line L748 (133.3599, 116.486) -> (126.4317, 104.486)
  line L749 (126.4317, 104.486) -> (133.3599, 92.486)
  line L750 (133.3599, 92.486) -> (147.2163, 92.486)
  line L751 (147.2163, 92.486) -> (154.1445, 104.486)
  line L752 (154.1445, 104.486) -> (147.2163, 116.486)
  line L753 (149.8143, 117.986) -> (156.7425, 105.986)
  line L754 (156.7425, 129.986) -> (149.8143, 117.986)
  line L755 (170.5989, 129.986) -> (156.7425, 129.986)
  line L756 (177.5272, 117.986) -> (170.5989, 129.986)
  line L757 (170.5989, 105.986) -> (177.5272, 117.986)
  line L758 (180.1252, 116.486) -> (173.197, 104.486)
  line L759 (156.7425, 105.986) -> (170.5989, 105.986)
  line L760 (170.5989, 102.986) -> (156.7425, 102.986)
  line L761 (177.5272, 90.986) -> (170.5989, 102.986)
  line L762 (170.5989, 78.986) -> (177.5272, 90.986)
  line L763 (156.7425, 78.986) -> (170.5989, 78.986)
  line L764 (149.8143, 90.986) -> (156.7425, 78.986)
  line L765 (156.7425, 102.986) -> (149.8143, 90.986)
  line L766 (193.9816, 116.486) -> (180.1252, 116.486)
  line L767 (173.197, 104.486) -> (180.1252, 92.486)
  line L768 (180.1252, 92.486) -> (193.9816, 92.486)
  line L769 (193.9816, 92.486) -> (200.9098, 104.486)
  line L770 (200.9098, 104.486) -> (193.9816, 116.486)
  line L771 (193.9816, 89.486) -> (180.1252, 89.486)
  line L772 (180.1252, 89.486) -> (173.197, 77.486)
  line L773 (173.197, 77.486) -> (180.1252, 65.486)
  line L774 (180.1252, 65.486) -> (193.9816, 65.486)
  line L775 (193.9816, 65.486) -> (200.9098, 77.486)
  line L776 (200.9098, 77.486) -> (193.9816, 89.486)
  line L777 (196.5797, 90.986) -> (203.5079, 78.986)
  line L778 (203.5079, 102.986) -> (196.5797, 90.986)
  line L779 (217.3643, 102.986) -> (203.5079, 102.986)
  line L780 (224.2925, 90.986) -> (217.3643, 102.986)
  line L781 (217.3643, 78.986) -> (224.2925, 90.986)
  line L782 (226.8906, 89.486) -> (219.9624, 77.486)
  line L783 (203.5079, 78.986) -> (217.3643, 78.986)
  line L784 (217.3643, 75.986) -> (203.5079, 75.986)
  line L785 (224.2925, 63.986) -> (217.3643, 75.986)
  line L786 (217.3643, 51.986) -> (224.2925, 63.986)
  line L787 (203.5079, 51.986) -> (217.3643, 51.986)
  line L788 (196.5797, 63.986) -> (203.5079, 51.986)
  line L789 (203.5079, 75.986) -> (196.5797, 63.986)
  line L790 (240.747, 89.486) -> (226.8906, 89.486)
  line L791 (219.9624, 77.486) -> (226.8906, 65.486)
  line L792 (226.8906, 65.486) -> (240.747, 65.486)
  line L793 (240.747, 65.486) -> (247.6752, 77.486)
  line L794 (247.6752, 77.486) -> (240.747, 89.486)
  line L795 (240.747, 62.486) -> (226.8906, 62.486)
  line L796 (226.8906, 62.486) -> (219.9624, 50.486)
  line L797 (219.9624, 50.486) -> (226.8906, 38.486)
  line L798 (226.8906, 38.486) -> (240.747, 38.486)
  line L799 (240.747, 38.486) -> (247.6752, 50.486)
  line L800 (247.6752, 50.486) -> (240.747, 62.486)
  line L801 (243.3451, 63.986) -> (250.2733, 51.986)
  line L802 (250.2733, 75.986) -> (243.3451, 63.986)
  line L803 (264.1297, 75.986) -> (250.2733, 75.986)
  line L804 (271.0579, 63.986) -> (264.1297, 75.986)
  line L805 (264.1297, 51.986) -> (271.0579, 63.986)
  line L806 (273.656, 62.486) -> (266.7278, 50.486)
  line L807 (250.2733, 51.986) -> (264.1297, 51.986)
  line L808 (264.1297, 48.986) -> (250.2733, 48.986)
  line L809 (271.0579, 36.986) -> (264.1297, 48.986)
  line L810 (264.1297, 24.986) -> (271.0579, 36.986)
  line L811 (250.2733, 24.986) -> (264.1297, 24.986)
  line L812 (243.3451, 36.986) -> (250.2733, 24.986)
  line L813 (250.2733, 48.986) -> (243.3451, 36.986)
  line L814 (287.5124, 62.486) -> (273.656, 62.486)
  line L815 (266.7278, 50.486) -> (273.656, 38.486)
  line L816 (273.656, 38.486) -> (287.5124, 38.486)
  line L817 (287.5124, 38.486) -> (294.4406, 50.486)
  line L818 (294.4406, 50.486) -> (287.5124, 62.486)
  line L819 (287.5124, 35.486) -> (273.656, 35.486)
  line L820 (273.656, 35.486) -> (266.7278, 23.486)
  line L821 (266.7278, 23.486) -> (273.656, 11.486)
  line L822 (273.656, 11.486) -> (287.5124, 11.486)
  line L823 (287.5124, 11.486) -> (294.4406, 23.486)
  line L824 (294.4406, 23.486) -> (287.5124, 35.486)
  line L825 (290.1105, 36.986) -> (297.0387, 24.986)
  line L826 (297.0387, 48.986) -> (290.1105, 36.986)
  line L827 (310.8951, 48.986) -> (297.0387, 48.986)
  line L828 (317.8233, 36.986) -> (310.8951, 48.986)
  line L829 (310.8951, 24.986) -> (317.8233, 36.986)
  line L830 (320.4213, 35.486) -> (313.4931, 23.486)
  line L831 (297.0387, 24.986) -> (310.8951, 24.986)
  line L832 (310.8951, 21.986) -> (297.0387, 21.986)
  line L833 (317.8233, 9.986) -> (310.8951, 21.986)
  line L834 (310.8951, -2.014) -> (317.8233, 9.986)
  line L835 (297.0387, -2.014) -> (310.8951, -2.014)
  line L836 (290.1105, 9.986) -> (297.0387, -2.014)
  line L837 (297.0387, 21.986) -> (290.1105, 9.986)
  line L838 (334.2777, 35.486) -> (320.4213, 35.486)
  line L839 (313.4931, 23.486) -> (320.4213, 11.486)
  line L840 (320.4213, 11.486) -> (334.2777, 11.486)
  line L841 (334.2777, 11.486) -> (341.206, 23.486)
  line L842 (341.206, 23.486) -> (334.2777, 35.486)
  line L843 (334.2777, 8.486) -> (320.4213, 8.486)
  line L844 (320.4213, 8.486) -> (313.4931, -3.514)
  line L845 (313.4931, -3.514) -> (320.4213, -15.514)
  line L846 (320.4213, -15.514) -> (334.2777, -15.514)
  line L847 (334.2777, -15.514) -> (341.206, -3.514)
  line L848 (341.206, -3.514) -> (334.2777, 8.486)
  line L849 (336.8758, 9.986) -> (343.804, -2.014)
  line L850 (343.804, 21.986) -> (336.8758, 9.986)
  line L851 (357.6604, 21.986) -> (343.804, 21.986)
  line L852 (364.5886, 9.986) -> (357.6604, 21.986)
  line L853 (357.6604, -2.014) -> (364.5886, 9.986)
  line L854 (367.1867, 8.486) -> (360.2585, -3.514)
  line L855 (343.804, -2.014) -> (357.6604, -2.014)
  line L856 (357.6604, -5.014) -> (343.804, -5.014)
  line L857 (364.5886, -17.014) -> (357.6604, -5.014)
  line L858 (357.6604, -29.014) -> (364.5886, -17.014)
  line L859 (343.804, -29.014) -> (357.6604, -29.014)
  line L860 (336.8758, -17.014) -> (343.804, -29.014)
  line L861 (343.804, -5.014) -> (336.8758, -17.014)
  line L862 (381.0431, 8.486) -> (367.1867, 8.486)
  line L863 (360.2585, -3.514) -> (367.1867, -15.514)
  line L864 (367.1867, -15.514) -> (381.0431, -15.514)
  line L865 (381.0431, -15.514) -> (387.9713, -3.514)
  line L866 (387.9713, -3.514) -> (381.0431, 8.486)
  line L867 (381.0431, -18.514) -> (367.1867, -18.514)
  line L868 (367.1867, -18.514) -> (360.2585, -30.514)
  line L869 (360.2585, -30.514) -> (367.1867, -42.514)
  line L870 (367.1867, -42.514) -> (381.0431, -42.514)
  line L871 (381.0431, -42.514) -> (387.9713, -30.514)
  line L872 (387.9713, -30.514) -> (381.0431, -18.514)
  line L873 (383.6412, -17.014) -> (390.5694, -29.014)
  line L874 (390.5694, -5.014) -> (383.6412, -17.014)
  line L875 (404.4258, -5.014) -> (390.5694, -5.014)
  line L876 (411.354, -17.014) -> (404.4258, -5.014)
  line L877 (404.4258, -29.014) -> (411.354, -17.014)
  line L878 (413.9521, -18.514) -> (407.0239, -30.514)
  line L879 (390.5694, -29.014) -> (404.4258, -29.014)
  line L880 (404.4258, -32.014) -> (390.5694, -32.014)
  line L881 (411.354, -44.014) -> (404.4258, -32.014)
  line L882 (404.4258, -56.014) -> (411.354, -44.014)
  line L883 (390.5694, -56.014) -> (404.4258, -56.014)
  line L884 (383.6412, -44.014) -> (390.5694, -56.014)
  line L885 (390.5694, -32.014) -> (383.6412, -44.014)
  line L886 (427.8085, -18.514) -> (413.9521, -18.514)
  line L887 (407.0239, -30.514) -> (413.9521, -42.514)
  line L888 (413.9521, -42.514) -> (427.8085, -42.514)
  line L889 (427.8085, -42.514) -> (434.7367, -30.514)
  line L890 (434.7367, -30.514) -> (427.8085, -18.514)
  line L891 (427.8085, -45.514) -> (413.9521, -45.514)
  line L892 (413.9521, -45.514) -> (407.0239, -57.514)
  line L893 (407.0239, -57.514) -> (413.9521, -69.514)
  line L894 (413.9521, -69.514) -> (427.8085, -69.514)
  line L895 (427.8085, -69.514) -> (434.7367, -57.514)
  line L896 (434.7367, -57.514) -> (427.8085, -45.514)
  line L897 (430.4066, -44.014) -> (437.3348, -56.014)
  line L898 (437.3348, -32.014) -> (430.4066, -44.014)
  line L899 (451.1912, -32.014) -> (437.3348, -32.014)
  line L900 (458.1194, -44.014) -> (451.1912, -32.014)
  line L901 (451.1912, -56.014) -> (458.1194, -44.014)
  line L902 (460.7175, -45.514) -> (453.7893, -57.514)
  line L903 (437.3348, -56.014) -> (451.1912, -56.014)
  line L904 (451.1912, -59.014) -> (437.3348, -59.014)
  line L905 (458.1194, -71.014) -> (451.1912, -59.014)
  line L906 (451.1912, -83.014) -> (458.1194, -71.014)